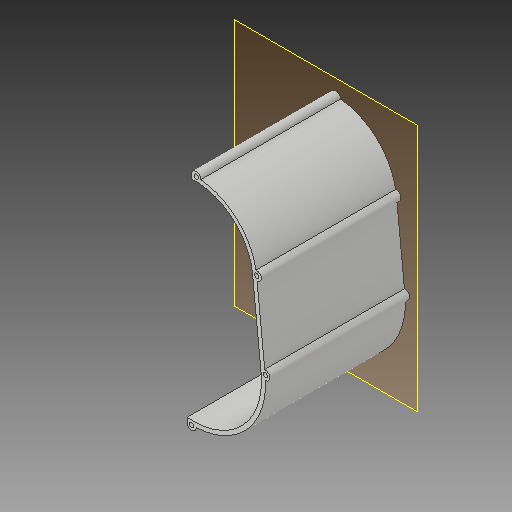
# Autodesk Inventor part: case bottom half
Saved by Autodesk Inventor 2017 (Build 210142000, 142)
## iProperties
Created: 2018-04-17
Part Number: case bottom half
Material: Generic
Document SubType Name: Modeling
Designer: RKL
Density: 1 g/cm^3
Appearance: Default
Author: RKL
Autodesk Inventor part; units mm, degrees
ref_plane "YZ Plane" through (0, 0, 0) normal (1, 0, 0) x (0, 1, 0)
ref_plane "XZ Plane" through (0, 0, 0) normal (0, 1, 0) x (-1, 0, 0)
ref_plane "XY Plane" through (0, 0, 0) normal (0, 0, 1) x (1, 0, 0)
ref_plane "Work Plane1" through (0, 0, 0) normal (0, 0, 1) x (1, 0, 0)
sketch "Sketch1" plane through (0, 0, 0) normal (0, 0, 1) x (1, 0, 0)
  circle A0 centre (-55.8916, -14.7421) radius 1.397 projected
  circle A1 centre (-83.8916, 18.2579) radius 1.397 projected
  circle A2 centre (-83.8916, -14.7421) radius 1.397 projected
  circle A3 centre (-55.8916, 18.2579) radius 1.397 projected
  circle A4 centre (2.1895, 105.4705) radius 2.159 projected
  circle A5 centre (-2.169, -104.4843) radius 2.159 projected
  circle A6 centre (60.6164, 51.7463) radius 2.159 projected
  circle A7 centre (-58.4167, 54.2173) radius 2.159 projected
  arc A8 (6.6818, 105.2084) -> (-2.3099, 105.3951) centre (2.1895, 105.4705) ccw projected
  arc A9 (-2.3099, 105.3951) -> (-57.5952, 58.6417) centre (0.9442, 45.4834) ccw construction
  arc A10 (-57.5952, 58.6417) -> (-59.0718, 49.7652) centre (-58.4167, 54.2173) ccw projected
  line L0 (-59.0718, 49.7652) -> (-63.1925, 21.7579) projected
  line L1 (-87.8916, 21.7579) -> (-63.1925, 21.7579) projected
  line L2 (-87.8916, -18.2421) -> (-87.8916, 21.7579) projected
  line L3 (-87.8916, -18.2421) -> (-74.0344, -26.2425) projected
  arc A11 (-74.0344, -26.2425) -> (-70.4822, -28.7807) centre (-69.9706, -24.3098) ccw projected
  arc A12 (-70.4822, -28.7807) -> (-6.6627, -104.2463) centre (-0.7162, -34.4994) ccw construction
  arc A13 (-6.6627, -104.2463) -> (2.3307, -104.433) centre (-2.169, -104.4843) ccw projected
  arc A14 (2.3307, -104.433) -> (69.2271, -31.6809) centre (-0.7162, -34.4994) ccw projected
  arc A15 (69.2271, -31.6809) -> (68.4317, -22.7173) centre (68.9014, -27.1927) ccw projected
  line L4 (68.4317, -22.7173) -> (61.0862, 47.2708) projected
  arc A16 (61.0862, 47.2708) -> (59.9792, 56.2009) centre (60.6164, 51.7463) ccw projected
  arc A17 (59.9792, 56.2009) -> (6.6818, 105.2084) centre (0.9442, 45.4834) ccw projected
  circle A18 centre (-69.9706, -24.3098) radius 2.159 projected
  circle A19 centre (68.9014, -27.1927) radius 2.159 projected
  circle A20 centre (0.9442, 45.4834) radius 17.5 projected
  circle A21 centre (-0.7162, -34.4994) radius 17.5 projected
  circle A22 centre (-66.7556, 10.6536) radius 4 projected
  circle A23 centre (-75.8916, -7.1378) radius 4 projected
  line L5 (-6.6627, -104.2463) -> (-2.3099, 105.3951) construction
  line L6 (-6.6627, -104.2463) -> (-6.5797, -100.2463)
  line L7 (-2.3099, 105.3951) -> (-2.393, 101.3951)
  arc A24 (-6.5797, -100.2463) -> (64.9314, -27.6121) centre (-0.7162, -34.4994) ccw
  arc A25 (56.6497, 51.3276) -> (-2.393, 101.3951) centre (0.9442, 45.4834) ccw
  line L8 (64.9314, -27.6121) -> (56.6497, 51.3276)
  point P0 (0, 0)
  dimension "d0" = 4
  dimension "d1" = 4
  constraints: 8 end point, 4 point on circle, 2 centre point, 2 coincident, 2 point on line, 2 tangent
  measures "d0" vertical distance of L5.end L7.end
  measures "d1" vertical distance of L5.start L6.end
extrude "Extrusion1" add sketch "Sketch1" along normal blind 135 contours A17 A16 L4 A15 A14 A13 L6 A24 L8 A25 L7 A8
body "Solid1"
